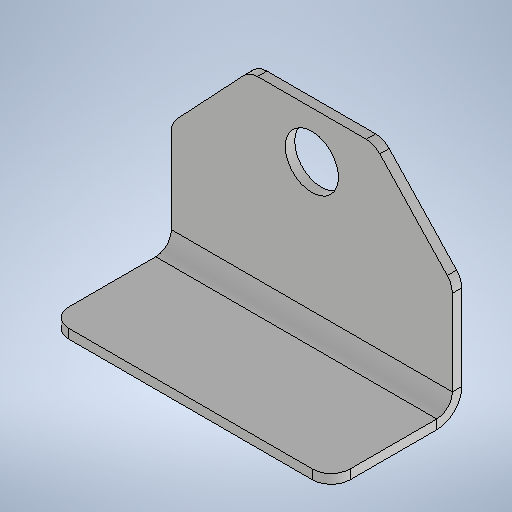
# Autodesk Inventor part: MSC 912 flange slipway
Saved by Autodesk Inventor 2025.1 (Build 291241020, 241B)
## iProperties
Created: 2024-07-01
Part Number: MSC 912 flange slipway
Material: Stainless Steel
Document SubType Name: Sheet Metal
Designer: admin
Stock Number: МОО 902 опора рамы
Mass: 530.491 g
Surface Area: 354.574 cm^2
Volume: 66.3114 cm^3
Density: 8 g/cm^3
Flat Pattern Width: 11.3388 cm
Flat Pattern Length: 11.4741 cm
Flat Pattern Area: 130.103 cm^2
Sheet Metal Rule: AISI304 3mm Die 32
Sheet Metal Width: 113.388 mm
Sheet Metal Length: 114.741 mm
Sheet Metal Area: 13010.302 mm^2
Appearance: Default
Author: pokla
Autodesk Inventor part; units mm, degrees
ref_plane "YZ Plane" through (0, 0, 0) normal (1, 0, 0) x (0, 1, 0)
ref_plane "XZ Plane" through (0, 0, 0) normal (0, 1, 0) x (-1, 0, 0)
ref_plane "XY Plane" through (0, 0, 0) normal (0, 0, 1) x (1, 0, 0)
sketch "Sketch1" plane through (0, 0, 0) normal (0, 1, 0) x (-1, 0, 0)
  line L0 (40, 40) -> (-40, 40) construction
  line L1 (-40, 40) -> (-40, -40) construction
  line L2 (-40, -40) -> (40, -40) construction
  line L3 (40, -40) -> (40, 40) construction
  line L4 (-40, 40) -> (40, -40) construction
  line L5 (100, -45) -> (-100, -45)
  line L6 (-100, -45) -> (-100, 100)
  line L7 (-100, 100) -> (100, 100)
  line L8 (100, 100) -> (100, -45)
  circle A0 centre (85, 0) radius 8.5
  circle A1 centre (0, 85) radius 8.5
  circle A2 centre (-85, 0) radius 8.5
  line L9 (0, 40) -> (0, -40) construction
  line L10 (100, 15) -> (20, 100)
  line L11 (-20, 100) -> (-100, 15)
  line L12 (100, -15) -> (71.7647, -45)
  line L13 (-100, -15) -> (-71.7647, -45)
  line L14 (0, 0) -> (-40, 0) construction
  line L15 (-45, -45) -> (-45, 73.4375)
  line L16 (45, -45) -> (45, 73.4375)
  line L17 (-45, 0) -> (45, 0)
  point P0 (0, 0)
  point P1 (0, 0)
  dimension "d2" = 80
  dimension "d3" = 80
  dimension "d17" = 5
  dimension "d18" = 17
  dimension "d19" = 45
  dimension "d20" = 45
  dimension "d21" = 40
  dimension "d22" = 15
  dimension "d23" = 15
  dimension "d24" = 30
  dimension "d26" = 5
  measures "d2" distance of L2.end L1.end
  measures "d3" distance of L1.end L0.end
  measures "d17" distance between parallel lines of L5 L2
  measures "d18" diameter of A1
  measures "d19" distance from line of A1.centre L0
  measures "d20" distance from line of L1 A2.centre
  measures "d21" distance of L11.start L10.end
  measures "d22" distance from line of L7 A1.centre
  measures "d23" distance from line of L6 A2.centre
  measures "d24" distance of L13.start L11.end
  measures "d26" distance between parallel lines of L1 L15
extrude "Plate1" add sketch "Sketch1" along normal blind 3 contours L17 L15 L11 L7 L10 L16
fillet "Corner Round5" radius 6 6 edges at (45, 1.5, 0) (-45, 1.5, 0) (45, 1.5, 73.4375) (20, 1.5, 100) (-20, 1.5, 100) (-45, 1.5, 73.4375)
sketch "Sketch3" plane through (0, 0, 0) normal (0, -1, 0) x (1, 0, 0)
  line L0 (39, 0) -> (-39, 0) projected
  line L1 (-45, 71.058) -> (-45, 6) projected
  line L2 (-45, 38.7474) -> (45, 38.7474)
  line L3 (45, 71.058) -> (45, 6) projected
  point P0 (0, 0)
  constraints: 2 end point, 2 point on line, 1 horizontal, 1 perpendicular
fold "Fold1" angle 90 bend radius 5 thickness 3 k factor 0.44 line from (-45, 0, 38.7474) to (45, 0, 38.7474) line at bend centre moving side (0, 0, -1) folds toward (0, -1, 0)
equation "\"d20\" = d19"
equation "\"d23\" = d22"
equation "\"d26\" = d17"
equation "\"d6\" = Thickness"
equation "\"d30\" = BendReliefWidth"
equation "\"d31\" = BendReliefDepth"
equation "\"d32\" = MinimumRemnant"
equation "\"d33\" = TransitionRadius"
equation "\"d35\" = BendRadius"
equation "\"BendReliefWidth\" = Thickness"
equation "\"BendReliefDepth\" = 0.5 * Thickness"
equation "\"CornerReliefSize\" = 4 * Thickness"
equation "\"MinimumRemnant\" = 2 * Thickness"
equation "\"TransitionRadius\" = BendRadius"
equation "\"JacobiRadiusSize\" = BendRadius"
equation "\"GapSize\" = Thickness"
equation "\"Thickness\" = 3"
equation "\"BendRadius\" = 5"
body "Solid1"
